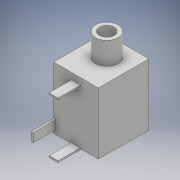
# Autodesk Inventor part: Parts_HLA-2503D1l
Saved by Autodesk Inventor 2018 (Build 220112000, 112)
## iProperties
Created: 2018-02-16
Part Number: Parts_HLA-2503D1l
Material: 一般
Document SubType Name: Modeling
Designer: sktom
Density: 1 g/cm^3
Appearance: 既定
Author: sktom
Autodesk Inventor part; units mm, degrees
ref_plane "YZ Plane" through (0, 0, 0) normal (1, 0, 0) x (0, 1, 0)
ref_plane "XZ Plane" through (0, 0, 0) normal (0, 1, 0) x (-1, 0, 0)
ref_plane "XY Plane" through (0, 0, 0) normal (0, 0, 1) x (1, 0, 0)
sketch "スケッチ1" plane through (0, 0, 0) normal (0, 0, 1) x (1, 0, 0)
  line L0 (-4, 4.5) -> (4, 4.5)
  line L1 (4, 4.5) -> (4, -4.5)
  line L2 (4, -4.5) -> (-4, -4.5)
  line L3 (-4, -4.5) -> (-4, 4.5)
  line L4 (-4, 4.5) -> (4, -4.5) construction
  line L5 (4, 4.5) -> (-4, -4.5) construction
  point P0 (0, 0)
  dimension "d0" = 8
  dimension "d1" = 9
  constraints: 12 end point, 2 midpoint, 2 parallel, 1 horizontal, 1 perpendicular
  measures "d0" distance of L0.start L0.end
  measures "d1" distance of L2.end L0.start
extrude "押し出し1" add sketch "スケッチ1" along normal blind 11
sketch "スケッチ2" plane through (0, 0, 11) normal (0, 0, 1) x (1, 0, 0)
  circle A0 centre (0, 1) radius 2
  circle A1 centre (0, 1) radius 1.3
  line L0 (-4, -4.5) -> (4, -4.5) projected
  point P0 (0, 0)
  dimension "d4" = 4
  dimension "d5" = 2.6
  dimension "d6" = 5.5
  constraints: 2 centre point, 1 coincident, 1 vertical alignment
  measures "d4" diameter of A0
  measures "d5" diameter of A1
  measures "d6" distance from line of L0 A0.centre
extrude "押し出し2" add sketch "スケッチ2" along normal blind 4
sketch "スケッチ3" plane through (-4, -4.5, 0) normal (0, -1, 0) x (1, 0, 0)
  line L0 (4.8, 9.85) -> (3.2, 9.85)
  line L1 (3.2, 9.85) -> (3.2, 9.55)
  line L2 (3.2, 9.55) -> (4.8, 9.55)
  line L3 (4.8, 9.55) -> (4.8, 9.85)
  line L4 (4.8, 9.85) -> (3.2, 9.55) construction
  line L5 (3.2, 9.85) -> (4.8, 9.55) construction
  line L6 (4.8, -0.15) -> (3.2, -0.15)
  line L7 (3.2, -0.15) -> (3.2, 0.15)
  line L8 (3.2, 0.15) -> (4.8, 0.15)
  line L9 (4.8, 0.15) -> (4.8, -0.15)
  line L10 (4.8, -0.15) -> (3.2, 0.15) construction
  line L11 (3.2, -0.15) -> (4.8, 0.15) construction
  line L12 (0, 11) -> (8, 11) projected
  line L13 (0.35, 2.3) -> (0.05, 2.3)
  line L14 (0.05, 2.3) -> (0.05, 0.7)
  line L15 (0.05, 0.7) -> (0.35, 0.7)
  line L16 (0.35, 0.7) -> (0.35, 2.3)
  line L17 (0.35, 2.3) -> (0.05, 0.7) construction
  line L18 (0.05, 2.3) -> (0.35, 0.7) construction
  point P0 (4, 0)
  point P1 (4, 9.7)
  point P2 (4, 9.7)
  point P3 (4, 0)
  point P4 (0.2, 1.5)
  dimension "d9" = 1.3
  dimension "d10" = 0.3
  dimension "d11" = 1.6
  dimension "d12" = 9.5
  dimension "d13" = 3.8
  constraints: 36 end point, 8 midpoint, 6 parallel, 4 equal length, 3 horizontal, 3 perpendicular, 1 vertical alignment
  measures "d9" distance from line of L12 point (4, 9.7)
  measures "d10" distance of L2.end L0.start
  measures "d11" distance of L1.end L2.end
  measures "d12" distance from line of L12 point (0.2, 1.5)
  measures "d13" horizontal distance of point (4, 0) point (0.2, 1.5)
extrude "押し出し3" add sketch "スケッチ3" along normal blind 4
